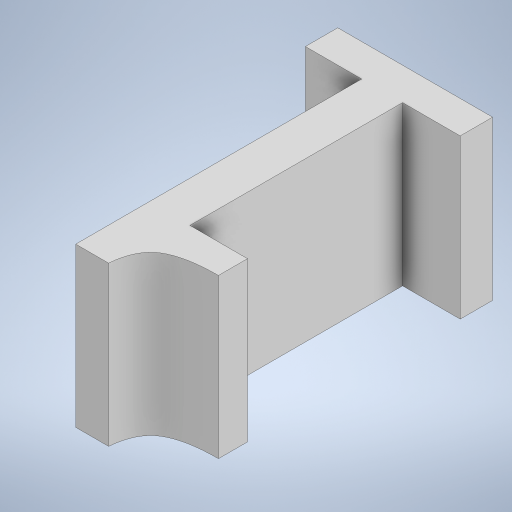
# Autodesk Inventor part: Text1
Saved by Autodesk Inventor 2023 (Build 270158000, 158)
## iProperties
Created: 2023-02-28
Part Number: Text1
Material: Generic
Document SubType Name: Modeling
Designer: 100KStarsun
Density: 1 g/cm^3
Appearance: Default
Author: 100KStarsun
Autodesk Inventor part; units mm, degrees
ref_plane "YZ Plane" through (0, 0, 0) normal (1, 0, 0) x (0, 1, 0)
ref_plane "XZ Plane" through (0, 0, 0) normal (0, 1, 0) x (-1, 0, 0)
ref_plane "XY Plane" through (0, 0, 0) normal (0, 0, 1) x (1, 0, 0)
sketch "Sketch1" plane through (0, 0, 0) normal (0, 1, 0) x (-1, 0, 0)
  line L0 (-3.8257, 4.2576) -> (4.1137, 4.2576) construction
  line L1 (4.1137, 4.2576) -> (4.1137, -4.4222) construction
  line L2 (4.1137, -4.4222) -> (-3.8257, -4.4222) construction
  line L3 (-3.8257, -4.4222) -> (-3.8257, 4.2576) construction
  line L4 (12.4147, -21.2247) -> (0.0234, -21.2247)
  line L5 (0.0234, -21.2247) -> (0.0234, -18.6312)
  line L6 (0.0234, -18.6312) -> (4.6341, -18.6312)
  line L7 (4.6341, -18.6312) -> (4.6341, -1.6087)
  line L8 (4.6341, -1.6087) -> (0.0234, -1.6087)
  line L9 (0.0234, -1.6087) -> (0.0234, 0.7173)
  spline S0 degree 2 poles (0.0234, 0.7173) (2.6375, 0.7173) (5.1075, 2.1993) (5.2722, 4.2576) knots 0 0 0 1 2 2 2
  line L10 (5.2722, 4.2576) -> (7.9069, 4.2576)
  line L11 (7.9069, 4.2576) -> (7.9069, -18.6312)
  line L12 (7.9069, -18.6312) -> (12.4147, -18.6312)
  line L13 (12.4147, -18.6312) -> (12.4147, -21.2247)
  point P0 (0, 0)
  constraints: 2 other
extrude "Extrusion1" add sketch "Sketch1" along normal blind 12.7
body "Solid1"
